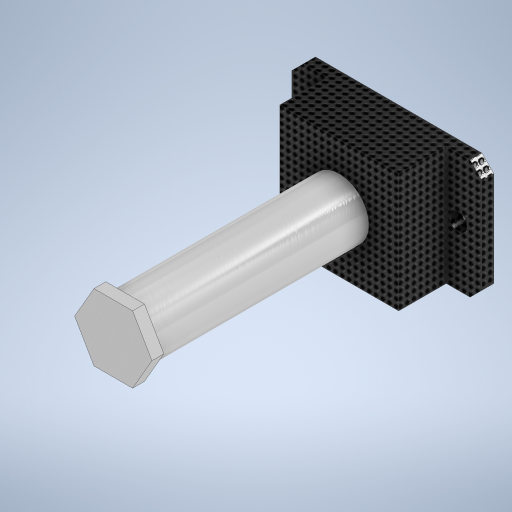
# Autodesk Inventor part: UpperArm
Saved by Autodesk Inventor 2024 (Build 280153000, 153)
## iProperties
Created: 2023-07-02
Part Number: UpperArm
Material: Generic
Document SubType Name: Modeling
Designer: vilas
Density: 1 g/cm^3
Appearance: Default
Author: vilas
Autodesk Inventor part; units mm, degrees
ref_plane "YZ Plane" through (0, 0, 0) normal (1, 0, 0) x (0, 1, 0)
ref_plane "XZ Plane" through (0, 0, 0) normal (0, 1, 0) x (-1, 0, 0)
ref_plane "XY Plane" through (0, 0, 0) normal (0, 0, 1) x (1, 0, 0)
sketch "Sketch1" plane through (0, 0, 0) normal (0, 0, 1) x (1, 0, 0)
  line L0 (-40, 25) -> (40, 25)
  line L1 (40, 25) -> (40, -25)
  line L2 (40, -25) -> (-40, -25)
  line L3 (-40, -25) -> (-40, 25)
  line L4 (-40, 25) -> (40, -25) construction
  line L5 (40, 25) -> (-40, -25) construction
  point P0 (0, 0)
  dimension "d0" = 80
  dimension "d1" = 50
  constraints: 12 end point, 2 midpoint, 2 parallel, 1 horizontal, 1 perpendicular
  measures "d0" distance of L1.end L2.end
  measures "d1" distance of L0.end L1.end
extrude "Extrusion1" add sketch "Sketch1" along normal blind 5
sketch "Sketch2" plane through (0, 0, 0) normal (0, 0, 1) x (1, 0, 0)
  line L0 (0, 0) -> (-30, 0) construction
  line L1 (0, 0) -> (30, 0) construction
  circle A0 centre (-30, 0) radius 3.75
  circle A1 centre (30, 0) radius 3.75
  dimension "d4" = 30
  dimension "d5" = 30
  dimension "d6" = 7.5
  dimension "d7" = 7.5
  constraints: 4 end point, 2 centre point, 2 coincident, 2 horizontal
  measures "d4" distance of L0.start L0.end
  measures "d5" distance of L0.start L1.end
  measures "d6" diameter of A0
  measures "d7" diameter of A1
extrude "Extrusion2" cut sketch "Sketch2" along normal through all
sketch "Sketch3" plane through (0, 0, 0) normal (0, 0, 1) x (1, 0, 0)
  line L0 (-25, 25) -> (25, 25)
  line L1 (25, 25) -> (25, -25)
  line L2 (25, -25) -> (-25, -25)
  line L3 (-25, -25) -> (-25, 25)
  line L4 (-25, 25) -> (25, -25) construction
  line L5 (25, 25) -> (-25, -25) construction
  point P0 (0, 0)
  dimension "d10" = 50
  dimension "d11" = 50
  constraints: 12 end point, 2 midpoint, 2 parallel, 1 horizontal, 1 perpendicular
  measures "d10" distance of L1.end L2.end
  measures "d11" distance of L0.end L1.end
extrude "Extrusion3" add sketch "Sketch3" along normal blind 25
sketch "Sketch4" plane through (0, 0, 25) normal (0, 0, 1) x (1, 0, 0)
  circle A0 centre (0, 0) radius 12.5
  dimension "d14" = 25
  constraints: 1 centre point, 1 coincident
  measures "d14" diameter of A0
extrude "Extrusion4" add sketch "Sketch4" along normal blind 90
sketch "Sketch5" plane through (0, 0, 115) normal (0, 0, 1) x (1, 0, 0)
  circle A0 centre (0, 0) radius 16.25 construction
  line L0 (16.25, 0) -> (8.125, -14.0729)
  line L1 (8.125, -14.0729) -> (-8.125, -14.0729)
  line L2 (-8.125, -14.0729) -> (-16.25, 0)
  line L3 (-16.25, 0) -> (-8.125, 14.0729)
  line L4 (-8.125, 14.0729) -> (8.125, 14.0729)
  line L5 (8.125, 14.0729) -> (16.25, 0)
  dimension "d17" = 32.5
  constraints: 12 end point, 2 coincident, 1 horizontal alignment, 15 other
extrude "Extrusion5" add sketch "Sketch5" along normal blind 5
chamfer "Chamfer1" distance 5 angle 45 4 edges at (40, -25, 2.5) (40, 25, 2.5) (-40, -25, 2.5) (-40, 25, 2.5)
body "Solid1"
